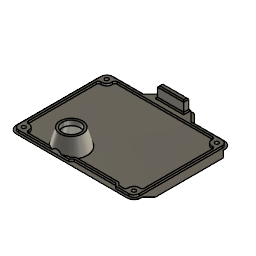
MainCaseTop (Autodesk Fusion 360 design; units mm, degrees)
Autodesk Fusion 360 part; units mm, degrees
sketch "Skizze1" plane through (0, 0, 0) normal (0, 0, 1) x (1, 0, 0)
  line L0 (50.5, -38) -> (-50.5, -38) construction
  line L1 (-50.5, -38) -> (-50.5, 38) construction
  line L2 (-50.5, 38) -> (50.5, 38) construction
  line L3 (50.5, 38) -> (50.5, -38) construction
  line L4 (50.5, -38) -> (-50.5, 38) construction
  line L5 (-50.5, -38) -> (50.5, 38) construction
  circle A0 centre (-50.5, 38) radius 4.8 construction
  circle A1 centre (-50.5, -38) radius 4.8 construction
  circle A2 centre (50.5, -38) radius 4.8 construction
  circle A3 centre (50.5, 38) radius 4.8 construction
  line L6 (-50.5, 45) -> (50.5, 45)
  line L7 (57.5, 38) -> (57.5, -38)
  line L8 (50.5, -45) -> (-50.5, -45)
  line L9 (-57.5, -38) -> (-57.5, 38)
  arc A4 (-50.5, 45) -> (-57.5, 38) centre (-50.5, 38) ccw
  arc A5 (-57.5, -38) -> (-50.5, -45) centre (-50.5, -38) ccw
  arc A6 (50.5, -45) -> (57.5, -38) centre (50.5, -38) ccw
  arc A7 (57.5, 38) -> (50.5, 45) centre (50.5, 38) ccw
  line L10 (-50.5, 42.8) -> (50.5, 42.8)
  line L11 (55.3, 38) -> (55.3, -38)
  line L12 (-55.3, -38) -> (-55.3, 38)
  line L13 (-53.3, 31.2472) -> (-53.3, -31.2472)
  line L14 (53.3, -31.2472) -> (53.3, 31.2472)
  line L15 (-43.7472, 40.8) -> (43.7472, 40.8)
  arc A8 (-51.0647, 33.2333) -> (-53.3, 31.2472) centre (-51.3, 31.2472) ccw
  arc A9 (-51.0647, 33.2333) -> (-45.7333, 38.5647) centre (-50.5, 38) ccw
  arc A10 (-43.7472, 40.8) -> (-45.7333, 38.5647) centre (-43.7472, 38.8) ccw
  arc A11 (50.5, -42.8) -> (55.3, -38) centre (50.5, -38) ccw
  arc A12 (55.3, 38) -> (50.5, 42.8) centre (50.5, 38) ccw
  arc A13 (-55.3, -38) -> (-50.5, -42.8) centre (-50.5, -38) ccw
  arc A14 (-50.5, 42.8) -> (-55.3, 38) centre (-50.5, 38) ccw
  arc A15 (45.7333, 38.5647) -> (43.7472, 40.8) centre (43.7472, 38.8) ccw
  arc A16 (45.7333, 38.5647) -> (51.0647, 33.2333) centre (50.5, 38) ccw
  arc A17 (53.3, 31.2472) -> (51.0647, 33.2333) centre (51.3, 31.2472) ccw
  arc A18 (43.7472, -40.8) -> (45.7333, -38.5647) centre (43.7472, -38.8) ccw
  arc A19 (51.0647, -33.2333) -> (45.7333, -38.5647) centre (50.5, -38) ccw
  arc A20 (51.0647, -33.2333) -> (53.3, -31.2472) centre (51.3, -31.2472) ccw
  arc A21 (-45.7333, -38.5647) -> (-43.7472, -40.8) centre (-43.7472, -38.8) ccw
  arc A22 (-45.7333, -38.5647) -> (-51.0647, -33.2333) centre (-50.5, -38) ccw
  arc A23 (-53.3, -31.2472) -> (-51.0647, -33.2333) centre (-51.3, -31.2472) ccw
  circle A24 centre (-50.5, -38) radius 1.75
  circle A25 centre (-50.5, 38) radius 1.75
  circle A26 centre (50.5, 38) radius 1.75
  circle A27 centre (50.5, -38) radius 1.75
  line L16 (-43.7472, -40.8) -> (-5.3284, -40.8)
  circle A28 centre (-15.5, -29.5) radius 8.25
  circle A29 centre (-15.5, -29.5) radius 10.25
  line L17 (57.5, 37) -> (63.5, 31)
  line L18 (63.5, 31) -> (63.5, -31)
  line L19 (63.5, -31) -> (57.5, -37)
  line L20 (-13, 42.8) -> (13, 42.8)
  line L21 (13, 42.8) -> (13, 51.8)
  line L22 (13, 51.8) -> (-13, 51.8)
  line L23 (-13, 51.8) -> (-13, 42.8)
  line L24 (-13, 51.8) -> (-22, 42.8)
  line L25 (13, 51.8) -> (22, 42.8)
  line L26 (-22.9113, 45) -> (-14.9113, 53)
  line L27 (-14.9113, 53) -> (14.9113, 53)
  line L28 (14.9113, 53) -> (22.9113, 45)
  line L29 (-12, 50.8) -> (12, 50.8)
  line L30 (12, 50.8) -> (12, 46)
  line L31 (12, 46) -> (-12, 46)
  line L32 (-12, 46) -> (-12, 50.8)
  line L33 (-50.5, -42.8) -> (-4.5, -42.8)
  line L34 (38.5, -42.8) -> (50.5, -42.8)
  line L35 (-4.5, -42.8) -> (-2, -40.3)
  line L36 (-2, -40.3) -> (36, -40.3)
  line L37 (36, -40.3) -> (38.5, -42.8)
  line L38 (-5.3284, -40.8) -> (-2.8284, -38.3)
  line L39 (-2.8284, -38.3) -> (36.8284, -38.3)
  line L40 (36.8284, -38.3) -> (39.3284, -40.8)
  line L41 (39.3284, -40.8) -> (43.7472, -40.8)
  point P0 (-15.5, -29.5)
  point P1 (38.5, -42.8)
  point P2 (-4.5, -42.8)
  dimension "d1" = 101
  dimension "d2" = 76
  dimension "d3" = 9.6
  dimension "d4" = 7
  dimension "d5" = 7
  dimension "d6" = 7
  dimension "d7" = 7
  dimension "d10" = 2
  dimension "d11" = 2
  dimension "d12" = 2
  dimension "d13" = 2
  dimension "d15" = 3.5
  dimension "d30" = 29.5
  dimension "d31" = 15.5
  dimension "d32" = 16.5
  dimension "d33" = 2
  dimension "d34" = 6
  dimension "d35" = 62
  dimension "d36" = 135
  dimension "d37" = 135
  dimension "d38" = 31
  dimension "d39" = 9
  dimension "d40" = 26
  dimension "d41" = 13
  dimension "d42" = 135
  dimension "d43" = 135
  dimension "d44" = 2.2
  dimension "d45" = 1.2
  dimension "d46" = 2.2
  dimension "d52" = 1
  dimension "d53" = 1
  dimension "d54" = 1
  dimension "d55" = 1
  dimension "d63" = 19
  dimension "d64" = 62
  dimension "d65" = 2.2
  dimension "d66" = 2.2
  dimension "d67" = 2.5
  dimension "d69" = 135
  dimension "d70" = 135
  dimension "d71" = 135
  dimension "d72" = 135
  dimension "d73" = 2
  dimension "d74" = 2
  dimension "d75" = 2
  dimension "d76" = 2
  constraint horizontal L0
  constraint perpendicular L0 L1
  constraint parallel L0 L2
  constraint parallel L1 L3
  constraint coincident L4 origin
  constraint coincident L5 origin
  constraint coincident L1.end L2.start
  constraint coincident L0.end L1.start
  constraint coincident L0.start L3.end
  constraint coincident L2.end L3.start
  constraint equal A0 A3
  constraint equal A0 A1
  constraint equal A1 A2
  constraint horizontal L6
  constraint vertical L7
  constraint horizontal L8
  constraint vertical L9
  constraint tangent L6 A4
  constraint tangent L9 A4
  constraint tangent L9 A5
  constraint tangent L8 A5
  constraint tangent L8 A6
  constraint tangent L7 A6
  constraint tangent L7 A7
  constraint tangent L6 A7
  constraint coincident A0 L10.start
  constraint coincident A3 L10.end
  constraint parallel L2 L10
  constraint coincident A3 L11.start
  constraint coincident A2 L11.end
  constraint perpendicular L10 L11
  constraint coincident A2 A11.start
  constraint coincident A1 A13.end
  constraint coincident A1 L12.start
  constraint coincident A0 L12.end
  constraint tangent A0 L12
  constraint tangent A0 L10
  constraint tangent A3 L11
  constraint parallel L1 L13
  constraint horizontal L16
  constraint vertical L14
  constraint horizontal L15
  constraint tangent L13 A8
  constraint tangent A8 A9
  constraint tangent A9 A10
  constraint coincident L15.start A10.start
  constraint tangent L15 A10
  constraint equal A0 A9
  constraint tangent L11 A12
  constraint tangent L12 A14
  constraint equal A8 A10
  constraint tangent L15 A15
  constraint tangent A15 A16
  constraint tangent A16 A17
  constraint equal A3 A16
  constraint equal A10 A15
  constraint equal A15 A17
  constraint tangent L14 A17
  constraint tangent A18 L16
  constraint tangent A18 A19
  constraint tangent A19 A20
  constraint equal A17 A20
  constraint equal A2 A19
  constraint equal A18 A20
  constraint coincident L14.start A20.end
  constraint tangent L14 A20
  constraint tangent A21 L16
  constraint tangent A21 A22
  constraint tangent A22 A23
  constraint equal A1 A22
  constraint equal A18 A21
  constraint equal A21 A23
  constraint tangent L13 A23
  constraint concentric A1 A24
  constraint concentric A4 A25
  constraint concentric A16 A26
  constraint concentric A6 A27
  constraint equal A24 A25
  constraint equal A25 A26
  constraint equal A26 A27
  constraint coincident P0 A28.centre
  constraint concentric A28 A29
  constraint parallel L7 L18
  constraint coincident L7 L19.end
  constraint coincident L7 L17.start
  constraint horizontal L20
  constraint vertical L21
  constraint horizontal L22
  constraint vertical L23
  constraint coincident L10 L20.start
  constraint coincident L10 L24.end
  constraint coincident L10 L25.end
  constraint coincident L6 L26.start
  constraint parallel L6 L27
  constraint coincident L6 L28.end
  constraint horizontal L29
  constraint vertical L30
  constraint horizontal L31
  constraint vertical L32
  constraint coincident P2 L33.end
  constraint tangent A1 L33
  constraint coincident P1 L34.start
  constraint tangent A2 L34
  constraint parallel L33 L36
  constraint parallel L16 L39
  constraint tangent A18 L41
  constraint tangent L12 A13
  constraint tangent L11 A11
  measures "d1" distance of L1.end L2.end
  measures "d2" distance of L0.end L1.end
  measures "d3" diameter of A0
  measures "d4" radius of A4
  measures "d5" radius of A5
  measures "d6" radius of A6
  measures "d7" radius of A7
  measures "d10" distance of L12 L13
  measures "d11" distance of L10 L15
  measures "d12" radius of A8
  measures "d13" distance of L11 L14
  measures "d15" diameter of A24
  measures "d30" vertical distance of origin A28.centre
  measures "d31" horizontal distance of origin P0
  measures "d32" diameter of A28
  measures "d33" distance of A28 A29
  measures "d34" distance of L7 L18
  measures "d35" distance of L17.end L18.end
  measures "d36" angle of L17 L18
  measures "d37" angle of L18 L19
  measures "d38" vertical distance of origin L17.end
  measures "d39" distance of L20.start L22.end
  measures "d40" distance of L21.end L22.end
  measures "d41" distance of origin L23
  measures "d42" angle of L22 L24
  measures "d43" angle of L22 L25
  measures "d44" distance of L24 L26
  measures "d45" distance of L22 L27
  measures "d46" distance of L25 L28
  measures "d52" distance of L21 L30
  measures "d53" distance of L23 L32
  measures "d54" distance of L22 L29
  measures "d55" distance of L6 L31
  measures "d63" distance of L7 P1
  measures "d64" distance of L7 P2
  measures "d65" distance of L8 L33
  measures "d66" distance of L8 L34
  measures "d67" distance of L34 L36
  measures "d69" angle of L36 L37
  measures "d70" angle of L35 L36
  measures "d71" angle of L39 L40
  measures "d72" angle of L38 L39
  measures "d73" distance of L35 L38
  measures "d74" distance of L37 L40
  measures "d75" distance of L34 L41
  measures "d76" distance of L36 L39
extrude "Extrusion1" add sketch "Skizze1" against normal blind 1 contours L6 L7 L8 L9 A4 A5 A6 A7 L10 L11 L12 A11 A12 A13 A14 L24 L25 L33 L34 L35 L36 L37 | L6 L22 L24 L25 L26 L27 L28 | L6 L23 L24 | L6 L10 L23 L24 | L6 L21 L22 L23 | L6 L10 L20 L21 L23 | L10 L11 L12 A11 A12 A13 A14 L20 L33 L34 L35 L36 L37 | L6 L21 L25 | L6 L10 L21 L25 | L7 L17 L18 L19 | L13 L14 L15 A8 A9 A10 A15 A16 A17 A18 A19 A20 A21 A22 A23 L16 L38 L39 L40 L41 | A29 | L29 L30 L31 L32
extrude "Extrusion2" add sketch "Skizze1" along normal blind 2 contours L6 L23 L24 | L6 L10 L23 L24 | L6 L21 L22 L23 | L6 L10 L20 L21 L23 | L10 L11 L12 A11 A12 A13 A14 L20 L33 L34 L35 L36 L37 | L6 L21 L25 | L6 L10 L21 L25 | L29 L30 L31 L32
extrude "Extrusion3" add sketch "Skizze1" along normal blind 15 contours A29
chamfer "Fase2" distance 1 angle 45 16 edges at (0, -45, -1) (55.4497, -42.9497, -1) (57.5, -37.5, -1) (-36.7056, 45, -1) (-55.4497, 42.9497, -1) (-57.5, 0, -1) (-55.4497, -42.9497, -1) (57.5, 37.5, -1) (55.4497, 42.9497, -1) (36.7056, 45, -1) (60.5, -34, -1) (63.5, 0, -1) (60.5, 34, -1) (-18.9113, 49, -1) (0, 53, -1) (18.9113, 49, -1)
draft "Verjüngung2" angle 16 neutral plane through (0, 0, 15) pull (0, 0, 1) 1 faces at (-5.3009, -30.5206, 10)
extrude "Extrusion4" cut sketch "Skizze1" along normal blind 10 contours L6 L7 L8 L9 A4 A5 A6 A7 L10 L11 L12 A11 A12 A13 A14 L24 L25 L33 L34 L35 L36 L37
extrude "Extrusion6" add sketch "Skizze1" along normal blind 12 contours L29 L30 L31 L32
chamfer "Fase3" distance 1 angle 45 8 edges at (12, 48.4, 2) (0, 46, 2) (0, 50.8, 2) (-12, 48.4, 2) (0, 46, 12) (12, 48.4, 12) (0, 50.8, 12) (-12, 48.4, 12)
chamfer "Fase4" distance 4 distance2 11.5 1 edges at (-23.1917, -32.4833, -1) measured on face at (30.1888, -8.2842, -1)
move_body "Verschieben1" bodies 1 to x (1, 0, 0) y (0, 1, 0) z (0, 0, 1) at (0, 0, 1)
equation "d59 = us_cone_diameter"
equation "d60 = us_cone_height"
equation "us_cone_diameter = 4 mm"
equation "us_cone_height = 11.5 mm"
